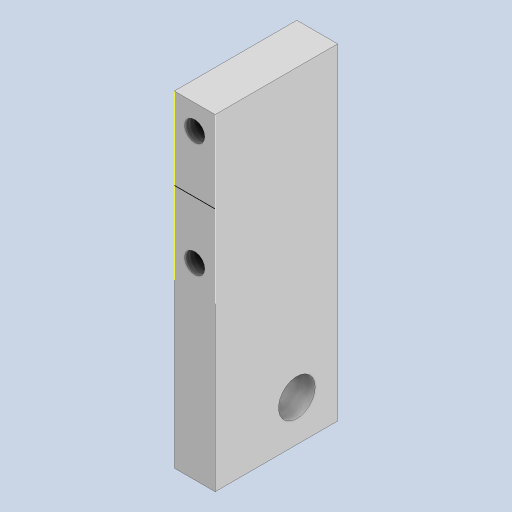
# Autodesk Inventor part: Al Attach block
Saved by Autodesk Inventor 2023.4 (Build 274418000, 418)
## iProperties
Created: 2024-01-12
Part Number: Al Attach block
Material: Generic
Document SubType Name: Modeling
Designer: PalumaCMM
Density: 1 g/cm^3
Appearance: Default
Author: PalumaCMM
Autodesk Inventor part; units mm, degrees
ref_plane "YZ Plane" through (0, 0, 0) normal (1, 0, 0) x (0, 1, 0)
ref_plane "XZ Plane" through (0, 0, 0) normal (0, 1, 0) x (-1, 0, 0)
ref_plane "XY Plane" through (0, 0, 0) normal (0, 0, 1) x (1, 0, 0)
sketch "Sketch1" plane through (0, 0, 0) normal (0, 0, 1) x (1, 0, 0)
  line L0 (0, 0) -> (5, 0)
  line L1 (5, 0) -> (5, 20)
  line L2 (5, 20) -> (0, 20)
  line L3 (0, 20) -> (0, 0)
  dimension "d0" = 5
  dimension "d1" = 20
  constraints: 8 end point, 2 parallel, 1 horizontal, 1 perpendicular
  measures "d0" distance of L2.end L1.end
  measures "d1" distance of L1.end L0.end
extrude "Extrusion1" add sketch "Sketch1" along normal blind 15
sketch "Sketch2" plane through (0, 0, 15) normal (0, 0, 1) x (1, 0, 0)
  line L0 (5, 20) -> (0, 20) projected
  circle A0 centre (2.5, 3) radius 1.5
  line L1 (0, 20) -> (0, 0) projected
  line L2 (0, 10) -> (5, 10)
  line L3 (5, 0) -> (5, 20) projected
  circle A1 centre (2.5, 17) radius 1.5
  line L4 (0, 0) -> (5, 0) projected
  point P0 (2.5, 0)
  dimension "d4" = 3
  dimension "d12" = 3
  constraints: 3 midpoint, 2 centre point, 2 end point, 1 symmetric about line, 1 other
  measures "d4" diameter of A0
  measures "d12" distance of point (2.5, 0) A0.centre
hole "Hole1" at (2.5, 17, 15) at (2.5, 3, 15) direction (0, 0, -1) diameter 2.459 end through all thread size "M3x0.5" class "6H" standard "ISO Metric profile"
sketch "Sketch3" plane through (0, 0, 15) normal (0, 0, 1) x (1, 0, 0)
  line L0 (0, 20) -> (0, 0) projected
  line L1 (0, 10) -> (5, 10)
  line L2 (5, 0) -> (5, 20) projected
  constraints: 2 end point, 2 midpoint
sketch "Sketch6" plane through (0, 0, 0) normal (-1, 0, 0) x (0, 0, 1)
  line L0 (0, 0) -> (0, 20) projected
  line L1 (0, 0) -> (15, 0)
  line L2 (15, 0) -> (15, -20)
  line L3 (15, -20) -> (0, -20)
  line L4 (0, -20) -> (0, 0)
  dimension "d24" = 15
  dimension "d25" = 20
  constraints: 8 end point, 2 parallel, 1 horizontal, 1 perpendicular
  measures "d24" distance of L2.end L3.end
  measures "d25" distance of L1.end L2.end
extrude "Extrusion2" add sketch "Sketch6" against normal blind 5
sketch "Sketch9" plane through (0, 20, 0) normal (-1, 0, 0) x (0, 0, 1)
  line L0 (0, -20) -> (15, -20)
  line L1 (15, 0) -> (15, -40) projected
  circle A0 centre (5, -35) radius 2.5
  line L2 (0, -40) -> (15, -40) projected
  line L3 (0, 0) -> (0, -40) projected
  point P0 (7.5, -40)
  dimension "d28" = 5
  dimension "d37" = 5
  dimension "d38" = 5
  constraints: 2 end point, 2 midpoint, 1 centre point, 1 horizontal
  measures "d28" diameter of A0
  measures "d37" distance from line of L3 A0.centre
  measures "d38" distance from line of L2 A0.centre
hole "Hole3" at (0, -15, 5) direction (1, 0, 0) diameter 4.5 end through all clearance for "Countersunk Flat Head Screw ISO 2009/7046" size "M4" standard "ISO"
body "Solid1"
